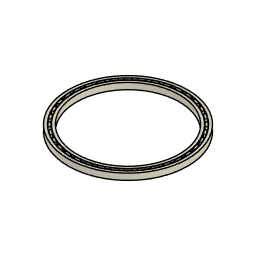
bearing_tutorial_195mm (Autodesk Fusion 360 design; units mm, degrees)
Autodesk Fusion 360 part; units mm, degrees
note: some values were not read from the file. Set by a fixed rule: which sketch regions a step uses.
sketch "Sketch1" plane through (0, 0, 0) normal (0, 0, 1) x (1, 0, 0)
  circle A0 centre (0, 0) radius 95
  circle A1 centre (0, 0) radius 90.6
  circle A2 centre (0, 0) radius 90.05
  circle A3 centre (0, 0) radius 86.65
  circle A4 centre (0, 0) radius 86.1
  circle A5 centre (0, 0) radius 81.7
  dimension "d1" = 190
  dimension "d2" = 4.4
  dimension "d3" = 0.55
  dimension "d4" = 3.4
  dimension "d5" = 0.55
  dimension "d6" = 4.4
  constraint coincident A0.centre A1.centre
  constraint concentric A0 A2
  constraint concentric A2 A3
  constraint concentric A2 A4
  constraint concentric A1 A5
  measures "d1" diameter of A0
  measures "d2" distance of A0 A1
  measures "d3" distance of A1 A2
  measures "d4" distance of A2 A3
  measures "d5" distance of A3 A4
  measures "d6" distance of A4 A5
extrude "Extrude1" add sketch "Sketch1" along normal blind 10 contours A0 makes body 1
extrude "Extrude2" add sketch "Sketch1" along normal blind 10 separate body contours A4 makes body 2
sketch "Sketch2" plane through (0, 0, 0) normal (0, 1, 0) x (1, 0, 0)
  line L0 (-95, -10) -> (95, -10) construction
  line L1 (90.6, -10) -> (-90.6, -10) construction
  line L2 (-86.1, -10) -> (86.1, -10) construction
  line L3 (81.7, -10) -> (-81.7, -10) construction
  line L4 (-95, 0) -> (95, 0) construction
  line L5 (86.1, -10) -> (86.1, 0) construction
  line L6 (90.6, -10) -> (90.6, 0) construction
  line L7 (90.6, -5) -> (86.1, -5) construction
  circle A0 centre (88.35, -5) radius 3.275
  dimension "d11" = 6.55
  constraint coincident L2.end L5.start
  constraint coincident L4 L5.end
  constraint perpendicular L4 L5
  constraint coincident L1.start L6.start
  constraint coincident L4 L6.end
  constraint perpendicular L4 L6
  constraint midpoint L6 L7.start
  constraint midpoint L5 L7.end
  constraint midpoint L7 A0.centre
  measures "d11" diameter of A0
revolve "Revolve1" cut sketch "Sketch2" angle 360 about axis through (0, 0, 1.75) along (0, 0, 1) bodies 1 2
extrude "Extrude3" add sketch "Sketch1" along normal blind 10 separate body contours A2 makes body 3
sketch "Sketch3" plane through (0, 0, 0) normal (0, 1, 0) x (1, 0, 0)
  line L0 (-90.05, -10) -> (90.05, -10) construction
  line L1 (0, 0) -> (0, -10) construction
  circle A0 centre (0, -5) radius 3.275
  line L2 (-3.175, -10) -> (-3.175, -5.8031)
  line L3 (3.175, -10) -> (3.175, -5.8031)
  line L4 (-3.175, -10) -> (3.175, -10)
  dimension "d15" = 6.55
  dimension "d16" = 3.175
  constraint coincident L1.start origin
  constraint midpoint L0 L1.end
  constraint midpoint L1 A0.centre
  constraint coincident L0 L2.start
  constraint coincident A0 L2.end
  constraint perpendicular L0 L2
  constraint symmetric L1 L2.start L3.start
  constraint symmetric L1 L2.end L3.end
  measures "d15" diameter of A0
  measures "d16" distance of L1 L2
extrude "Extrude4" cut sketch "Sketch3" along normal through all bodies 3
pattern_circular "C-Pattern1" count 36 over 360 about axis through (0, 0, 1.75) along (0, 0, 1) of "Extrude4"
sketch "Sketch4" plane through (0, 0, 0) normal (0, 1, 0) x (1, 0, 0)
  line L0 (-86.1, -10) -> (86.1, -10) construction
  line L1 (90.6, -10) -> (-90.6, -10) construction
  line L2 (-95, 0) -> (95, 0) construction
  line L3 (86.1, -10) -> (86.1, 0) construction
  line L4 (90.6, -10) -> (90.6, 0) construction
  line L5 (86.1, -5) -> (90.6, -5) construction
  circle A0 centre (88.35, -5) radius 3.175
  line L6 (88.35, -5) -> (88.35, -8.175)
  line L7 (88.35, -5) -> (88.35, -1.825)
  dimension "d20" = 6.35
  constraint coincident L0.end L3.start
  constraint coincident L2 L3.end
  constraint perpendicular L2 L3
  constraint coincident L1.start L4.start
  constraint coincident L2 L4.end
  constraint perpendicular L2 L4
  constraint midpoint L3 L5.start
  constraint midpoint L4 L5.end
  constraint midpoint L5 A0.centre
  constraint coincident A0.centre L6.start
  constraint coincident A0 L6.end
  constraint perpendicular L5 L6
  constraint coincident A0 L7.end
  constraint perpendicular L5 L7
  measures "d20" diameter of A0
revolve "Revolve2" add sketch "Sketch4" angle 360 about axis through (88.35, 0, 5) along (0, 0, 1) separate body contours A0 L6 L7 picked at (88.7988, -7.063) makes body 4
pattern_circular "C-Pattern2" count 36 over 360 about axis through (0, 0, 1.75) along (0, 0, 1) of bodies 4 makes body 5 at (88.0844, 18.2998, 5.4144) makes body 6 at (82.4752, 27.1175, 5.4144) makes body 7 at (76.5133, 47.3228, 5.4144) makes body 8 at (64.722, 57.8669, 5.4144) makes body 9 at (55.7137, 70.638, 5.4144) makes body 10 at (47.3228, 76.5133, 4.5856) makes body 11 at (29.1409, 80.0638, 4.5856) makes body 12 at (14.7952, 83.9078, 4.5856) makes body 13 at (-2.7261, 89.9239, 4.5856) makes body 14 at (-17.7532, 84.9844, 5.4144) makes body 15 at (-27.1175, 82.4752, 4.5856) makes body 16 at (-47.3228, 76.5133, 5.4144) makes body 17 at (-57.8669, 64.722, 5.4144) makes body 18 at (-70.638, 55.7137, 5.4144) makes body 19 at (-76.5133, 41.0272, 5.4144) makes body 20 at (-80.6105, 32.2409, 4.5856) makes body 21 at (-88.0844, 18.2998, 4.5856) makes body 22 at (-89.9239, 2.7261, 4.5856) makes body 23 at (-83.9078, -14.7952, 5.4144) makes body 24 at (-82.4752, -27.1175, 5.4144) makes body 25 at (-76.5133, -41.0272, 5.4144) makes body 26 at (-64.722, -57.8669, 5.4144) makes body 27 at (-55.7137, -70.638, 5.4144) makes body 28 at (-47.3228, -76.5133, 5.4144) makes body 29 at (-33.3175, -83.5685, 5.4144) makes body 30 at (-18.2998, -88.0844, 4.5856) makes body 31 at (-2.7261, -89.9239, 4.5856) makes body 32 at (14.7952, -83.9078, 5.4144) makes body 33 at (27.1175, -82.4752, 5.4144) makes body 34 at (47.3228, -76.5133, 5.4144) makes body 35 at (55.7137, -70.638, 5.4144) makes body 36 at (70.638, -55.7137, 5.4144) makes body 37 at (76.5133, -47.3228, 4.5856) makes body 38 at (83.5685, -33.3175, 4.5856) makes body 39 at (84.9844, -17.7532, 5.4144)
equation "d11 = ( 25.4 / 4 ) * 1 mm + 0.2 mm"
equation "d15 = ( 25.4 / 4 ) * 1 mm + 0.2 mm"
equation "d16 = ( 25.4 / 4 / 2 ) * 1 mm"
equation "d20 = ( 25.4 / 4 ) * 1 mm"
named bodies: "outer", "inner", "middle"
